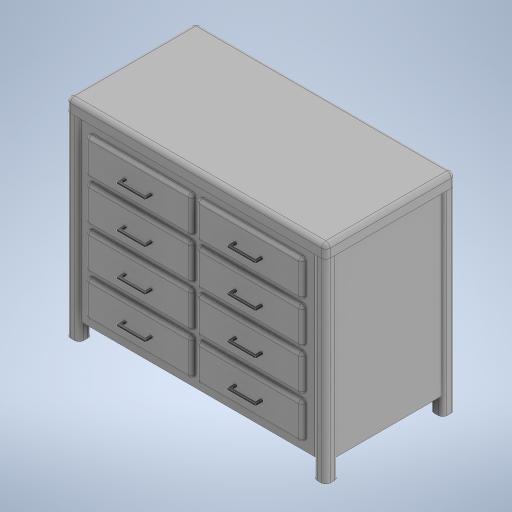
# Autodesk Inventor part: Dresser Configurator
Saved by Autodesk Inventor 2023 (Build 270158000, 158)
## iProperties
Company: Jay's Dressers
RuleStatus: InUse
Created: 2022-06-23
Part Number: Dresser Configurator
Material: Generic
Document SubType Name: Modeling
Designer: Admin
Density: 1 g/cm^3
Appearance: Default
dresserHeight: 48.000 in
topThickness: 3.000 in
dresserWidth: 60.000 in
drawerRows: 4.000 ul
drawerColumns: 2.000 ul
panelThickness: 1.000 in
drawerHeight: 6.500 in
drawerVerticalOffset: 3.000 in
drawerWidth: 22.500 in
drawerHorizontalOffset: 3.000 in
dresserDepth: 30.000 in
Author: Cadflair
Title: Dresser Configurator
Autodesk Inventor part; units mm, degrees
sketch "Base Sketch" plane through (0, 0, 0) normal (0, 1, 0) x (-1, 0, 0)
  line L0 (-762, 381) -> (762, 381) construction
  line L1 (762, 381) -> (762, -381) construction
  line L2 (762, -381) -> (-762, -381) construction
  line L3 (-762, -381) -> (-762, 381) construction
  line L4 (-762, 381) -> (762, -381) construction
  line L5 (762, 381) -> (-762, -381) construction
  line L6 (762, 381) -> (685.8, 381)
  line L7 (685.8, 381) -> (685.8, 304.8)
  line L8 (685.8, 304.8) -> (762, 304.8)
  line L9 (762, 304.8) -> (762, 381)
  line L10 (-762, 381) -> (-685.8, 381)
  line L11 (-685.8, 381) -> (-685.8, 304.8)
  line L12 (-685.8, 304.8) -> (-762, 304.8)
  line L13 (-762, 304.8) -> (-762, 381)
  line L14 (-762, -381) -> (-685.8, -381)
  line L15 (-685.8, -381) -> (-685.8, -304.8)
  line L16 (-685.8, -304.8) -> (-762, -304.8)
  line L17 (-762, -304.8) -> (-762, -381)
  line L18 (762, -381) -> (685.8, -381)
  line L19 (685.8, -381) -> (685.8, -304.8)
  line L20 (685.8, -304.8) -> (762, -304.8)
  line L21 (762, -304.8) -> (762, -381)
  point P0 (0, 0)
  dimension "dresserWidth" = 1524
  dimension "dresserDepth" = 762
  dimension "legDepth" = 76.2
  dimension "legWidth" = 76.2
  constraints: 44 end point, 10 parallel, 5 equal length, 5 horizontal, 5 perpendicular, 2 midpoint, 1 point on line
  measures "dresserWidth" distance of L1.end L2.end
  measures "dresserDepth" distance of L0.end L1.end
  measures "legDepth" distance of L6.end L7.end
  measures "legWidth" distance of L7.end L8.end
ref_plane "Top Plane" through (0, 1219.2, 0) normal (0, 1, 0) x (-1, 0, 0)
sketch "Top Sketch" plane through (0, 1219.2, 0) normal (0, 1, 0) x (-1, 0, 0)
  line L0 (762, 381) -> (762, -381) projected
  line L1 (762, -381) -> (-762, -381) projected
  line L2 (-762, 381) -> (762, 381) projected
  line L3 (-762, -381) -> (-762, 381) projected
  point P0 (0, 0)
ref_plane "Front Plane" through (0, 0, 342.9) normal (0, 0, 1) x (1, 0, 0)
sketch "Front Panel Sketch" plane through (0, 0, 342.9) normal (0, 0, 1) x (1, 0, 0)
  line L0 (685.8, 101.6) -> (-685.8, 101.6)
  line L1 (-685.8, 101.6) -> (-685.8, 1143)
  line L2 (-685.8, 1143) -> (685.8, 1143)
  line L3 (685.8, 1143) -> (685.8, 101.6)
  line L4 (762, 1219.2) -> (-762, 1219.2) construction
  point P0 (0, 0)
  point P1 (0, 101.6)
  point P2 (-685.8, 0)
  point P3 (-685.8, 0)
  point P4 (-685.8, 0)
  point P5 (685.8, 0)
  point P6 (685.8, 0)
  point P7 (685.8, 0)
  dimension "legExposure" = 101.6
  dimension "d7" = 76.2
  dimension "frontPanelWidth" = 1371.6
  dimension "frontPanelHeight" = 1041.4
  constraints: 8 end point, 3 vertical alignment, 2 parallel, 1 horizontal, 1 midpoint, 1 perpendicular
  measures "legExposure" distance from line of point (0, 0) L0
  measures "d7" distance between parallel lines of L2 L4
  measures "frontPanelWidth" distance of L0.start L0.end
  measures "frontPanelHeight" distance of L0.end L1.end
sketch "Drawer Cut Sketch" plane through (0, 0, 342.9) normal (0, 0, 1) x (1, 0, 0)
  line L0 (-685.8, 101.6) -> (-685.8, 1143) construction
  line L1 (685.8, 101.6) -> (-685.8, 101.6) construction
  line L2 (-609.6, 177.8) -> (-38.1, 177.8)
  line L3 (-38.1, 177.8) -> (-38.1, 342.9)
  line L4 (-38.1, 342.9) -> (-609.6, 342.9)
  line L5 (-609.6, 342.9) -> (-609.6, 177.8)
  line L6 (-12.7, 368.3) -> (-12.7, 152.4)
  line L7 (-12.7, 152.4) -> (-635, 152.4)
  line L8 (-635, 152.4) -> (-635, 368.3)
  line L9 (-635, 368.3) -> (-12.7, 368.3)
  point P0 (0, 0)
  dimension "drawerHeight" = 165.1
  dimension "drawerVerticalOffset" = 76.2
  dimension "drawerWidth" = 571.5
  dimension "drawerHorizontalOffset" = 76.2
  dimension "d37" = 25.4
  constraints: 16 end point, 4 parallel, 2 perpendicular, 1 horizontal, 3 other
  measures "drawerHeight" distance of L4.end L2.start
  measures "drawerVerticalOffset" distance between parallel lines of L5 L0
  measures "drawerWidth" distance of L3.end L4.end
  measures "drawerHorizontalOffset" distance between parallel lines of L2 L1
  measures "d37" distance between parallel lines of L3 L6
ref_plane "Back Plane" through (0, 0, -342.9) normal (0, 0, 1) x (1, 0, 0)
sketch "Back Panel Sketch" plane through (0, 0, -342.9) normal (0, 0, 1) x (1, 0, 0)
  line L0 (685.8, 1143) -> (685.8, 101.6) projected
  line L1 (-685.8, 1143) -> (685.8, 1143) projected
  line L2 (685.8, 101.6) -> (-685.8, 101.6) projected
  line L3 (-685.8, 101.6) -> (-685.8, 1143) projected
  point P0 (0, 0)
ref_plane "Right Plane" through (723.9, 0, 0) normal (1, 0, 0) x (0, 1, 0)
ref_plane "Left Plane" through (-723.9, 0, 0) normal (1, 0, 0) x (0, 1, 0)
sketch "Right Panel Sketch" plane through (723.9, 0, 0) normal (1, 0, 0) x (0, 1, 0)
  line L0 (1143, -342.9) -> (101.6, -342.9) projected
  line L1 (1143, 342.9) -> (101.6, 342.9) projected
  line L2 (1143, 342.9) -> (1143, -342.9)
  line L3 (101.6, -342.9) -> (101.6, 342.9)
  point P0 (0, 0)
  constraints: 4 end point, 1 parallel, 1 perpendicular
sketch "Left Panel Sketch" plane through (-723.9, 0, 0) normal (1, 0, 0) x (0, 1, 0)
  line L0 (101.6, -342.9) -> (1143, -342.9) projected
  line L1 (101.6, 342.9) -> (1143, 342.9) projected
  line L2 (101.6, -342.9) -> (101.6, 342.9)
  line L3 (1143, -342.9) -> (1143, 342.9)
  point P0 (0, 0)
  constraints: 4 end point, 1 perpendicular, 1 vertical
extrude "Front Panel Extrusion" add sketch "Front Panel Sketch" along normal blind 25.4
extrude "Right Panel Extrusion" add sketch "Right Panel Sketch" along normal blind 25.4
extrude "Left Panel Extrusion" add sketch "Left Panel Sketch" against normal blind 25.4
extrude "Rear Panel Extrusion" add sketch "Back Panel Sketch" against normal blind 25.4
extrude "Drawer Cutout Extrusion" cut sketch "Drawer Cut Sketch" along normal up to surface (25.4 mm away) contours L5 L4 L3 L2
extrude "Drawer Face Extrusion" add sketch "Drawer Cut Sketch" along normal blind 25.4 from surface at 25.4 contours L5 L4 L3 L2 | L6 L7 L8 L9
fillet "Drawer Fillet1" radius 19.05 8 edges at (-635, 368.3, 381) (-323.85, 368.3, 393.7) (-635, 260.35, 393.7) (-12.7, 368.3, 381) (-12.7, 260.35, 393.7) (-323.85, 152.4, 393.7) (-12.7, 152.4, 381) (-635, 152.4, 381)
pattern_linear "Drawer Rectangular Pattern" count 2 spacing 647.7 along (1, 0, 0) count 4 spacing 241.3 along (0, 1, 0) of "Drawer Cutout Extrusion", "Drawer Face Extrusion", "Drawer Fillet1"
ref_plane "Drawer Mid Plane1" through (-615.95, 260.35, 374.65) normal (0, 1, 0) x (1, 0, 0)
sketch "Sketch11" plane through (-615.95, 260.35, 374.65) normal (0, 1, 0) x (1, 0, 0)
  line L0 (0, -19.05) -> (584.2, -19.05) projected
  line L1 (209.55, -19.05) -> (374.65, -19.05)
  line L2 (374.65, -19.05) -> (374.65, -63.5)
  line L3 (374.65, -63.5) -> (209.55, -63.5)
  line L4 (209.55, -63.5) -> (209.55, -19.05)
  line L5 (222.25, -19.05) -> (222.25, -50.8)
  line L6 (222.25, -50.8) -> (361.95, -50.8)
  line L7 (361.95, -50.8) -> (361.95, -19.05)
  point P0 (615.95, 374.65)
  point P1 (292.1, -19.05)
  point P2 (374.65, -19.05)
  dimension "d68" = 44.45
  dimension "d69" = 165.1
  dimension "d70" = 12.7
  dimension "d71" = 12.7
  dimension "d72" = 12.7
  constraints: 14 end point, 3 perpendicular, 2 midpoint, 2 parallel, 2 point on line, 1 horizontal, 1 vertical
  measures "d68" distance of L3.end L1.start
  measures "d69" distance of L2.end L3.end
  measures "d70" distance between parallel lines of L5 L4
  measures "d71" distance between parallel lines of L2 L7
  measures "d72" distance between parallel lines of L6 L3
extrude "Square Handle Extrusion" add sketch "Sketch11" along normal mid plane 12.7 separate body contours L0 L5 L6 L7 L2 L3 L4
ref_plane "Drawer Mid Plane2" through (-323.85, 171.45, 374.65) normal (1, 0, 0) x (0, 0, -1)
sketch "Sketch10" plane through (-323.85, 171.45, 374.65) normal (1, 0, 0) x (0, 0, -1)
  line L0 (-19.05, 0) -> (-19.05, 177.8) projected
  line L1 (-19.05, 93.6625) -> (-19.05, 88.9)
  line L2 (-19.05, 88.9) -> (-57.15, 88.9)
  arc A0 (-44.45, 114.3) -> (-57.15, 88.9) centre (-25.4, 88.9) ccw
  line L3 (-44.45, 114.3) -> (-41.275, 114.3)
  line L4 (-41.275, 114.3) -> (-41.275, 93.6625)
  line L5 (-41.275, 93.6625) -> (-19.05, 93.6625)
  point P0 (374.65, -171.45)
  dimension "d61" = 38.1
  dimension "d62" = 3.175
  dimension "d63" = 22.225
  dimension "d64" = 9.525
  dimension "d65" = 50.8
  constraints: 10 end point, 3 perpendicular, 2 point on circle, 1 centre point, 1 midpoint, 1 parallel, 1 point on line, 1 vertical
  measures "d61" distance of L1.end L2.end
  measures "d62" distance of L3.start L3.end
  measures "d63" distance of L4.end L1.start
  measures "d64" diameter of L5 L2
  measures "d65" diameter of L3 L2
revolve "Round Knob Revolution1" add sketch "Sketch10" angle 360 about axis through (-323.85, 260.35, 393.7) along (0, 0, 1) separate body
fillet "Round Knob Fillet" radius 0.635 2 edges at (-323.85, 234.95, 419.1) (-323.85, 234.95, 415.925)
sketch "Sketch8" plane through (-323.85, 171.45, 374.65) normal (1, 0, 0) x (0, 0, -1)
  line L0 (-19.05, 101.6) -> (-19.05, 76.2)
  line L1 (-19.05, 76.2) -> (-44.45, 76.2)
  arc A0 (-19.05, 101.6) -> (-44.45, 76.2) centre (-19.05, 76.2) ccw
  line L2 (-19.05, 0) -> (-19.05, 177.8) projected
  point P0 (374.65, -171.45)
  point P1 (-19.05, 88.9)
  dimension "d43" = 25.4
  constraints: 4 end point, 2 midpoint, 2 perpendicular, 2 point on circle, 1 centre point, 1 point on line, 1 vertical
  measures "d43" distance of L0.end L1.end
extrude "Bin Pull Exrusion" add sketch "Sketch8" along normal mid plane 127 separate body
fillet "Bin Pull Fillet" radius 25.4 2 edges at (-387.35, 265.6105, 411.6605) (-260.35, 265.6105, 411.6605)
sketch "Sketch9" plane through (-260.35, 247.65, 393.7) normal (0, 0, -1) x (-1, 0, 0)
  arc A0 (25.4, 25.4) -> (0, 0) centre (25.4, 0) ccw projected
  line L0 (127, 0) -> (0, 0) projected
  arc A1 (127, 0) -> (101.6, 25.4) centre (101.6, 0) ccw projected
  line L1 (101.6, 25.4) -> (25.4, 25.4) projected
  arc A2 (25.4, 28.575) -> (-2.9981, -3.175) centre (25.4, 0) ccw
  line L2 (-2.9981, -3.175) -> (129.9981, -3.175)
  arc A3 (129.9981, -3.175) -> (101.6, 28.575) centre (101.6, 0) ccw
  line L3 (101.6, 28.575) -> (25.4, 28.575)
  line L4 (0, 0) -> (-3.175, 0)
  line L5 (127, 0) -> (130.175, 0)
  point P0 (-260.35, -247.65)
  dimension "d47" = 3.175
  constraints: 8 end point, 6 point on circle, 2 centre point, 2 horizontal, 3 other
  measures "d47" distance between parallel lines of L1 L3
extrude "Bin Pull Exrusion2" add sketch "Sketch9" against normal blind 3.175 contours A0 L4 A2 L3 A3 L5 A1 L1 bodies 4
pattern_linear "Handle Rectangular Pattern" count 2 spacing 647.7 along (1, 0, 0) count 4 spacing 241.3 along (0, 1, 0) bodies 4 3 2
extrude "Top Extrusion" add sketch "Top Sketch" against normal blind 76.2 bodies 1
fillet "Fillet3" radius 25.4 8 edges at (-762, 1181.1, 381) (-762, 1219.2, 0) (0, 1219.2, 381) (762, 1181.1, 381) (762, 1219.2, 0) (0, 1219.2, -381) (-762, 1181.1, -381) (762, 1181.1, -381)
extrude "Leg Extrusion" add sketch "Base Sketch" along normal up to surface (1143 mm away) separate body
fillet "Leg Fillet" radius 25.4 16 edges at (-685.8, 571.5, 304.8) (-685.8, 571.5, 381) (-762, 571.5, 381) (-762, 571.5, 304.8) (-762, 571.5, -304.8) (-685.8, 571.5, -304.8) (-762, 571.5, -381) (-685.8, 571.5, -381) (685.8, 571.5, -381) (685.8, 571.5, -304.8) (762, 571.5, -381) (762, 571.5, -304.8) (762, 571.5, 304.8) (762, 571.5, 381) (685.8, 571.5, 381) (685.8, 571.5, 304.8)
equation "\"d7\" = topThickness"
equation "\"d17\" = panelThickness"
equation "\"d19\" = panelThickness"
equation "\"d21\" = panelThickness"
equation "\"d23\" = panelThickness"
equation "\"d25\" = panelThickness"
equation "\"d38\" = panelThickness"
equation "\"d29\" = drawerWidth + drawerVerticalOffset"
equation "\"d32\" = drawerHeight + drawerHorizontalOffset"
equation "\"d71\" = d70"
equation "\"d72\" = d70"
equation "\"d33\" = topThickness"
equation "\"d52\" = d29"
equation "\"d55\" = d32"
equation "\"topThickness\" = 76.2"
equation "\"d5\" = 0.5 * dresserDepth - 0.5 * legDepth"
equation "\"drawerRows\" = 4"
equation "\"drawerColumns\" = 2"
equation "\"panelThickness\" = 25.4"
equation "\"d14\" = -0.5 * dresserDepth + 0.5 * legDepth"
equation "\"d15\" = 0.5 * dresserWidth - 0.5 * legWidth"
equation "\"d16\" = -0.5 * dresserWidth + 0.5 * legWidth"
